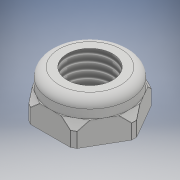
# Autodesk Inventor part: nut
Saved by Autodesk Inventor 2017 SP1 (Build 210196100, 196)
## iProperties
Part Number: nut
Material: 一般
Document SubType Name: Modeling
Designer: gisen
Density: 1 g/cm^3
Appearance: 既定
Author: gisen
Autodesk Inventor part; units mm, degrees
note: some values were not read from the file. Chosen so that the rebuilt part matches the saved one: second side of "押し出し1".
ref_plane "YZ Plane" through (0, 0, 0) normal (1, 0, 0) x (0, 1, 0)
ref_plane "XZ Plane" through (0, 0, 0) normal (0, 1, 0) x (-1, 0, 0)
ref_plane "XY Plane" through (0, 0, 0) normal (0, 0, 1) x (1, 0, 0)
sketch "スケッチ1" plane through (0, 0, 0) normal (0, 0, 1) x (1, 0, 0)
  line L0 (8, 0) -> (4, 6.9282)
  line L1 (4, 6.9282) -> (-4, 6.9282)
  line L2 (-4, 6.9282) -> (-8, 0)
  line L3 (-8, 0) -> (8, 0)
  line L4 (-8, 0) -> (-4, -6.9282)
  line L5 (-8, 0) -> (0, 0) construction
  line L6 (-4, -6.9282) -> (4, -6.9282)
  line L7 (4, -6.9282) -> (8, 0)
  point P0 (0, 0)
  point P1 (0, 0)
  dimension "d0" = 8
  dimension "d2" = 8
  dimension "d3" = 8
  dimension "d4" = 8
  dimension "d5" = 60
  dimension "d6" = 8
  dimension "d7" = 60
  dimension "d9" = 8
  constraints: 16 end point, 3 horizontal, 1 coincident, 1 equal length, 1 midpoint
  measures "d0" distance of L0.start L0.end
  measures "d2" distance of L0.end L1.end
  measures "d3" distance of L1.end L2.end
  measures "d4" distance of L2.end L4.end
  measures "d5" angle of L4 L5
  measures "d6" distance of L4.end L6.end
  measures "d7" angle of L2 L3
  measures "d9" distance of L6.end L0.start
extrude "押し出し1" add sketch "スケッチ1" against normal blind 4
sketch "スケッチ5" plane through (0, 0, 0) normal (0, 0, 1) x (1, 0, 0)
  circle A0 centre (0, 0) radius 6.9282
  line L0 (-4, -6.9282) -> (4, -6.9282) projected
  line L1 (4, 6.9282) -> (-4, 6.9282) projected
  dimension "d38" = 13.8564
  dimension "d39" = 13.8564
  constraints: 1 centre point, 1 coincident
  measures "d38" diameter of A0
  measures "d39" distance between parallel lines of L0 L1
extrude "押し出し2" add sketch "スケッチ5" along normal blind 3
sketch "スケッチ4" plane through (0, 0, -4) normal (0, 0, -1) x (1, 0, 0)
  point P0 (0, 0)
  point P1 (0, 0)
  constraints: 1 coincident
hole "穴3" at (0, 0, -4) direction (0, 0, 1) diameter 8 end through all
fillet "フィレット1" radius 1.5 1 edges at (-6.9282, 0, 3)
chamfer "面取り1" distance 0.5 angle 45 6 edges at (4, 6.9282, -2) (-4, 6.9282, -2) (8, 0, -2) (-8, 0, -2) (-4, -6.9282, -2) (4, -6.9282, -2)
sketch "スケッチ6" plane through (0, 0, 0) normal (0, 1, 0) x (-1, 0, 0)
  line L0 (-6.9282, 0) -> (-6.9282, 1.5) projected
  line L1 (-7.75, 0) -> (-6, 0) projected
  line L2 (-6.9282, 0) -> (-7.75, -1.4234)
  line L3 (-6.9282, 0) -> (-5.2846, 0) construction
  line L4 (-7.75, -4) -> (-7.75, 0) projected
  line L5 (-6, 0) -> (-7.75, 0) projected
  line L6 (-7.75, -1.4234) -> (-7.75, 0)
  line L7 (-7.75, 0) -> (-6.9282, 0)
  point P0 (0, 0)
  dimension "d44" = 120
  constraints: 8 end point, 1 equal length, 1 horizontal, 1 perpendicular, 1 point on line, 1 vertical
  measures "d44" angle of L2 L3
extrude "押し出し3" cut sketch "スケッチ6" along normal through all both and the other way through all
pattern_circular "円形状パターン1" count 6 over 360 about axis through (0, 0, 18.2935) along (0, 0, -1) of "押し出し3"
fillet "フィレット2" radius 0.1 5 edges at (2.6782, -6.9282, -0.7117) (3.5, -6.9282, -2.7117) (4.25, -6.4952, -2.7117) (4.6609, -5.7835, -0.7117) (3.875, -6.7117, -1.4234)
pattern_circular "円形状パターン2" count 6 over 360 about axis through (0, 0, 18.2935) along (0, 0, -1) of "フィレット2"
thread "ねじ1" size "M8x1.25" class "6H" standard "ANSI Metric M Profile" full length
equation "\"d38\" = d39"
